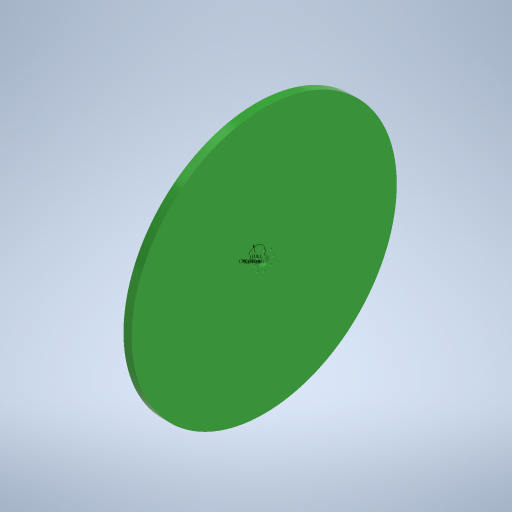
# Autodesk Inventor part: uMule-kolo_napędowe
Saved by Autodesk Inventor 2024.2 (Build 282272000, 272)
## iProperties
Created: 2024-10-21
Part Number: uMule-kolo_napędowe
Material: Ogólny
Document SubType Name: Modeling
Designer: owozn
Density: 1 g/cm^3
Appearance: Domyślna
Author: owozn
Autodesk Inventor part; units mm, degrees
ref_plane "YZ Plane" through (0, 0, 0) normal (1, 0, 0) x (0, 1, 0)
ref_plane "XZ Plane" through (0, 0, 0) normal (0, 1, 0) x (-1, 0, 0)
ref_plane "XY Plane" through (0, 0, 0) normal (0, 0, 1) x (1, 0, 0)
sketch "Szkic1" plane through (0, 0, 0) normal (0, 0, 1) x (1, 0, 0)
  line L0 (-41.2071, 0) -> (178.5929, 0) projected
  line L1 (0, -47.06) -> (0, 194.51) projected
  line L2 (0, 0) -> (0, 6) construction
  line L3 (0, 6) -> (-4.1, 6)
  line L4 (-4.1, 6) -> (-4.8071, 5.2929)
  line L5 (-4.1, 6) -> (-3.1, 6) construction
  line L6 (0, 0) -> (-4.8071, 0) construction
  line L7 (-4.8071, 0) -> (-4.8071, 3) construction
  line L8 (-4.8071, 3) -> (-4.8071, 5.2929)
  line L9 (-4.8071, 3) -> (-9.8071, 3)
  line L10 (-9.8071, 3) -> (-9.8071, 160)
  line L11 (-9.8071, 3) -> (147.1929, 3) construction
  line L12 (-9.8071, 160) -> (0, 160)
  line L13 (0, 160) -> (0, 6)
  dimension "d0" = 6
  dimension "d1" = 4.1
  dimension "d5" = 1
  dimension "d6" = 135
  dimension "d7" = 3
  dimension "d8" = 5
  dimension "d9" = 157
  dimension "d10" = 90
  constraints: 24 end point, 4 horizontal, 3 point on line, 3 vertical, 2 equal length, 1 collinear, 1 perpendicular
  measures "d0" distance of L2.start L2.end
  measures "d1" distance of L2.end L3.end
  measures "d5" distance of L3.end L4.end
  measures "d6" angle of L4 L5
  measures "d7" distance of L6.end L7.end
  measures "d8" distance of L7.end L9.end
  measures "d9" distance of L9.end L10.end
  measures "d10" angle of L11 L10
revolve "Obrót1" add sketch "Szkic1" angle 360 about axis through (-10, 0, 0) along (1, 0, 0)
sketch "Szkic2" plane through (-9.8071, 0, 0) normal (-1, 0, 0) x (0, 0, 1)
  line L0 (0, 0) -> (11, 0) construction
  circle A0 centre (11, 0) radius 1.55
  circle A1 centre (7.7782, 7.7782) radius 1.55
  circle A2 centre (0, 11) radius 1.55
  circle A3 centre (-7.7782, 7.7782) radius 1.55
  circle A4 centre (-11, 0) radius 1.55
  circle A5 centre (-7.7782, -7.7782) radius 1.55
  circle A6 centre (0, -11) radius 1.55
  circle A7 centre (7.7782, -7.7782) radius 1.55
  circle A8 centre (0, 0) radius 14
  circle A9 centre (0, 0) radius 5.05
  line L1 (5.8312, 0) -> (2.9156, -5.05)
  line L2 (2.9156, 5.05) -> (5.8312, 0)
  line L3 (-2.9156, 5.05) -> (2.9156, 5.05)
  line L4 (-5.8312, 0) -> (-2.9156, 5.05)
  line L5 (-2.9156, -5.05) -> (-5.8312, 0)
  line L6 (2.9156, -5.05) -> (-2.9156, -5.05)
  point P0 (0, -5.05)
  dimension "d21" = 10.1
  dimension "d12" = 11
  dimension "d13" = 3.1
  dimension "d16" = 360
  dimension "d20" = 28
  dimension "d26" = 360
  constraints: 14 end point, 9 centre point, 4 coincident, 1 horizontal, 1 point on line, 1 vertical alignment, 39 other
  measures "d12" distance of L0.start L0.end
  measures "d13" diameter of A0
  measures "d20" diameter of A8
extrude "Wyciągnięcie proste1" cut sketch "Szkic2" against normal through all contours A0 | A1 | A2 | A3 | A4 | A5 | A6 | A7
extrude "Wyciągnięcie proste2" add sketch "Szkic2" along normal blind 10
fillet "Zaokrąglenie1" radius 10 1 edges at (-9.8071, 0, -14)
